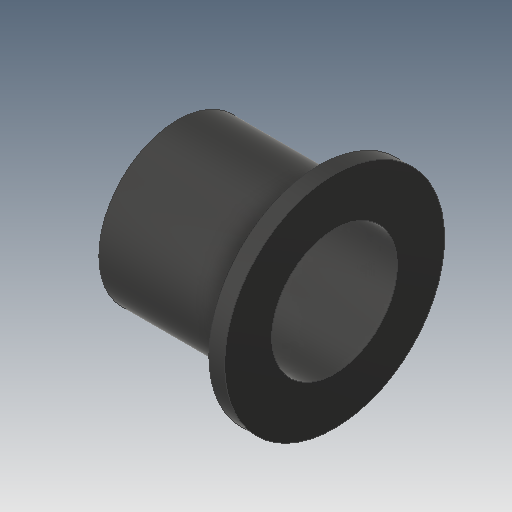
# Autodesk Inventor part: p8-10_OilessFlange
Saved by Autodesk Inventor 2019.4 (Build 234330000, 330)
## iProperties
Created: 2019-06-14
Part Number: p8-10_OilessFlange
Material: アセタール樹脂、黒
Document SubType Name: Modeling
Designer: AzLIer
Density: 1.425 g/cm^3
Appearance: 滑らか - 黒
Mass: 0.510352 g
Surface Area: 7.85398 cm^2
Volume: 0.358142 cm^3
Author: AzLIer
Autodesk Inventor part; units mm, degrees
ref_plane "YZ Plane" through (0, 0, 0) normal (1, 0, 0) x (0, 1, 0)
ref_plane "XZ Plane" through (0, 0, 0) normal (0, 1, 0) x (-1, 0, 0)
ref_plane "XY Plane" through (0, 0, 0) normal (0, 0, 1) x (1, 0, 0)
sketch "スケッチ1" plane through (0, 0, 0) normal (1, 0, 0) x (0, 1, 0)
  circle A0 centre (0, 0) radius 5
  circle A1 centre (0, 0) radius 4
  dimension "d0" = 10
  dimension "d1" = 8
  constraints: 2 centre point, 2 coincident
  measures "d0" diameter of A0
  measures "d1" diameter of A1
extrude "押し出し1" add sketch "スケッチ1" along normal blind 10
sketch "スケッチ2" plane through (10, 0, 0) normal (1, 0, 0) x (0, 0, -1)
  circle A0 centre (0, 0) radius 4 projected
  circle A1 centre (0, 0) radius 7
  dimension "d4" = 14
  constraints: 1 centre point, 1 coincident
  measures "d4" diameter of A1
extrude "押し出し2" add sketch "スケッチ2" against normal blind 1
